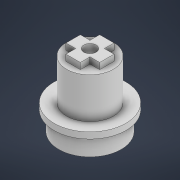
# Autodesk Inventor part: Motor_Servo_Welle_Test
Saved by Autodesk Inventor 2021 (Build 250183000, 183)
## iProperties
Created: 2021-01-21
Part Number: Motor_Servo_Welle_Test
Material: Generisch
Document SubType Name: Modeling
Designer: Ctroi
Density: 1 g/cm^3
Appearance: Vorgabe
Author: Ctroi
Autodesk Inventor part; units mm, degrees
ref_plane "YZ Plane" through (0, 0, 0) normal (1, 0, 0) x (0, 1, 0)
ref_plane "XZ Plane" through (0, 0, 0) normal (0, 1, 0) x (-1, 0, 0)
ref_plane "XY Plane" through (0, 0, 0) normal (0, 0, 1) x (1, 0, 0)
sketch "Skizze1" plane through (0, 0, 0) normal (0, 1, 0) x (-1, 0, 0)
  circle A0 centre (0, 0) radius 10
  dimension "d0" = 20
  constraints: 1 centre point, 1 coincident
  measures "d0" diameter of A0
extrude "Extrusion1" add sketch "Skizze1" along normal blind 6
sketch "Skizze2" plane through (0, 6, 0) normal (0, 1, 0) x (1, 0, 0)
  circle A0 centre (0, 0) radius 11.5
  dimension "d3" = 23
  constraints: 1 centre point, 1 coincident
  measures "d3" diameter of A0
extrude "Extrusion2" add sketch "Skizze2" along normal blind 2
sketch "Skizze3" plane through (0, 8, 0) normal (0, 1, 0) x (1, 0, 0)
  circle A0 centre (0, 0) radius 7.5
  dimension "d6" = 15
  constraints: 1 centre point, 1 coincident
  measures "d6" diameter of A0
extrude "Extrusion3" add sketch "Skizze3" along normal blind 13
sketch "Skizze4" plane through (0, 21, 0) normal (0, 1, 0) x (1, 0, 0)
  line L0 (-5.4, 5.4) -> (5.4, 5.4)
  line L1 (5.4, 5.4) -> (5.4, -5.4)
  line L2 (5.4, -5.4) -> (-5.4, -5.4)
  line L3 (-5.4, -5.4) -> (-5.4, 5.4)
  line L4 (0, 16.1) -> (0, -16.1) projected
  line L5 (-16.1, 0) -> (16.1, 0) projected
  line L6 (-5.4, 5.4) -> (-2.3, 5.4)
  line L7 (-2.3, 5.4) -> (-2.3, 2.3)
  line L8 (-2.3, 2.3) -> (-5.4, 2.3)
  line L9 (-5.4, 2.3) -> (-5.4, 5.4)
  line L10 (5.4, 5.4) -> (2.3, 5.4)
  line L11 (2.3, 5.4) -> (2.3, 2.3)
  line L12 (2.3, 2.3) -> (5.4, 2.3)
  line L13 (5.4, 2.3) -> (5.4, 5.4)
  line L14 (5.4, -5.4) -> (2.3, -5.4)
  line L15 (2.3, -5.4) -> (2.3, -2.3)
  line L16 (2.3, -2.3) -> (5.4, -2.3)
  line L17 (5.4, -2.3) -> (5.4, -5.4)
  line L18 (-5.4, -5.4) -> (-2.3, -5.4)
  line L19 (-2.3, -5.4) -> (-2.3, -2.3)
  line L20 (-2.3, -2.3) -> (-5.4, -2.3)
  line L21 (-5.4, -2.3) -> (-5.4, -5.4)
  point P0 (0, 0)
  point P1 (5.4, 2.3)
  point P2 (-5.4, 2.3)
  point P3 (-5.4, -2.3)
  point P4 (2.3, -5.4)
  point P5 (5.4, -2.3)
  dimension "d9" = 10.8
  dimension "d10" = 10.8
  dimension "d11" = 3.1
  dimension "d12" = 3.1
  dimension "d13" = 3.1
  dimension "d14" = 3.1
  dimension "d15" = 3.1
  dimension "d16" = 3.1
  dimension "d17" = 3.1
  dimension "d18" = 3.1
  constraints: 40 end point, 10 parallel, 5 horizontal, 5 perpendicular, 2 other
  measures "d9" distance of L1.end L2.end
  measures "d10" distance of L0.end L1.end
  measures "d11" distance of L7.end L8.end
  measures "d12" distance of L6.end L7.end
  measures "d13" distance of L12.end L11.end
  measures "d14" distance of L11.end L10.end
  measures "d15" distance of L15.end L16.end
  measures "d16" distance of L14.end L15.end
  measures "d17" distance of L20.end L19.end
  measures "d18" distance of L19.end L18.end
extrude "Extrusion4" add sketch "Skizze4" along normal blind 2 contours L0 L4 L5 L3 L8 L7 | L0 L11 L12 L1 L5 L4 | L5 L4 L2 L19 L20 L3 | L5 L1 L16 L15 L2 L4
sketch "Skizze5" plane through (0, 23, 0) normal (0, 1, 0) x (1, 0, 0)
  circle A0 centre (0, 0) radius 2
  dimension "d21" = 4
  constraints: 1 centre point, 1 coincident
  measures "d21" diameter of A0
extrude "Extrusion5" cut sketch "Skizze5" against normal blind 5
